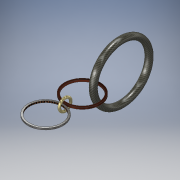
# Autodesk Inventor part: 4 ring revolve
Saved by Autodesk Inventor 2017 (Build 210142000, 142)
## iProperties
Created: 2018-09-17
Part Number: 4 ring revolve
Material: Generic
Document SubType Name: Modeling
Designer: qthuynh
Density: 1 g/cm^3
Appearance: Default
Author: qthuynh
Autodesk Inventor part; units mm, degrees
ref_plane "XY Plane" through (0, 0, 0) normal (0, 0, 1) x (1, 0, 0)
sketch "Sketch1" plane through (0, 0, 0) normal (0, 1, 0) x (-1, 0, 0)
  circle A0 centre (0, 0) radius 4.7986
  line L0 (-3.1183, -22.2001) -> (2.8357, -22.2001)
  constraints: 2 end point, 1 centre point, 1 coincident, 1 horizontal
revolve "Revolution1" add sketch "Sketch1" angle 360 about axis through (3.1183, 0, -22.2001) along (-1, 0, 0)
ref_plane "Work Plane1" through (0, 0, 0) normal (1, 0, 0) x (0, 1, 0)
ref_plane "Work Plane2" through (0, 0, 0) normal (0, 1, 0) x (-1, 0, 0)
sketch "Sketch2" plane through (0, 0, 0) normal (1, 0, 0) x (0, 1, 0)
  line L0 (-1.4768, -19.8879) -> (5.415, -19.8879)
  line L1 (5.415, -19.8879) -> (5.415, -27.0751)
  line L2 (5.415, -27.0751) -> (-1.4768, -27.0751)
  line L3 (-1.4768, -27.0751) -> (-1.4768, -19.8879)
  line L4 (-10.6503, -89.4076) -> (11.1118, -89.4076)
  point P0 (0, 0)
  constraints: 10 end point, 2 horizontal, 2 parallel, 1 perpendicular
revolve "Revolution2" add sketch "Sketch2" angle 360 about axis through (0, -10.6503, -89.4076) along (0, 1, 0)
sketch "Sketch3" plane through (0, 0, 0) normal (0, 1, 0) x (-1, 0, 0)
  ellipse E0 centre (0, -131.9928) end of major axis (-12.9123, -131.9928) minor radius 11.4829
  line L0 (6.6953, -240.0739) -> (-12.9123, -240.0739)
  point P0 (0, 0)
  constraints: 2 end point, 1 horizontal, 2 other
revolve "Revolution3" add sketch "Sketch3" angle 360 about axis through (-6.6953, 0, -240.0739) along (1, 0, 0)
sketch "Sketch4" plane through (0, 0, 0) normal (1, 0, 0) x (0, 1, 0)
  line L0 (0, -8.6325) -> (6.1825, -8.6325)
  line L1 (6.1825, -8.6325) -> (6.1825, -14.9313)
  line L2 (6.1825, -14.9313) -> (0, -14.9313)
  line L3 (0, -14.9313) -> (0, -8.6325)
  line L4 (-4.6514, 53.3472) -> (6.1825, 53.3472)
  point P0 (0, 0)
  constraints: 10 end point, 2 horizontal, 2 parallel, 1 perpendicular
revolve "Revolution4" add sketch "Sketch4" angle 360 about axis through (0, -4.6514, 53.3472) along (0, 1, 0)
mirror "Mirror1" about plane through (0, 0, 0) normal (0, 1, 0) of "Revolution3"
body "Solid1"
